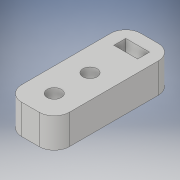
# Autodesk Inventor part: Gantry_simplified
Saved by Autodesk Inventor 2018 (Build 220112000, 112)
## iProperties
Created: 2020-03-14
Part Number: Gantry_simplified
Material: Generic
Document SubType Name: Modeling
Designer: natha
Density: 1 g/cm^3
Appearance: Default
Author: natha
Autodesk Inventor part; units mm, degrees
ref_plane "YZ Plane" through (0, 0, 0) normal (1, 0, 0) x (0, 1, 0)
ref_plane "XZ Plane" through (0, 0, 0) normal (0, 1, 0) x (-1, 0, 0)
ref_plane "XY Plane" through (0, 0, 0) normal (0, 0, 1) x (1, 0, 0)
sketch "Sketch1" plane through (0, 0, 0) normal (0, 1, 0) x (-1, 0, 0)
  line L0 (0, 0) -> (40, 0)
  line L1 (40, 0) -> (40, -100)
  line L2 (40, -100) -> (0, -100)
  line L3 (0, -100) -> (0, 0)
  circle A0 centre (20, -20) radius 6
  circle A1 centre (20, -50) radius 6
  line L4 (30, -80) -> (10, -80)
  line L5 (10, -80) -> (10, -90)
  line L6 (10, -90) -> (30, -90)
  line L7 (30, -90) -> (30, -80)
  dimension "d0" = 40
  dimension "d1" = 100
  dimension "d2" = 12
  dimension "d3" = 12
  dimension "d4" = 20
  dimension "d5" = 20
  dimension "d6" = 30
  dimension "d7" = 20
  dimension "d8" = 20
  dimension "d9" = 10
  dimension "d10" = 10
  dimension "d11" = 10
  constraints: 16 end point, 4 parallel, 2 centre point, 2 horizontal, 2 perpendicular
  measures "d0" distance of L1.end L2.end
  measures "d1" distance of L0.end L1.end
  measures "d2" diameter of A0
  measures "d3" diameter of A1
  measures "d4" distance from line of L3 A1.centre
  measures "d5" distance from line of L3 A0.centre
  measures "d6" distance of A1.centre A0.centre
  measures "d7" distance from line of L0 A0.centre
  measures "d8" distance of L6.end L5.end
  measures "d9" distance of L5.end L4.end
  measures "d10" distance between parallel lines of L3 L5
  measures "d11" distance between parallel lines of L2 L6
extrude "Extrusion1" add sketch "Sketch1" along normal blind 25
fillet "Fillet1" radius 12.7 4 edges at (0, 12.5, -100) (0, 12.5, 0) (-40, 12.5, 0) (-40, 12.5, -100)
body "Solid1"
